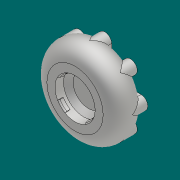
# Autodesk Inventor part: finger5
Saved by Autodesk Inventor 2018.2 (Build 222227000, 227)
## iProperties
Created: 2020-12-02
Part Number: finger5
Material: アルミニウム 6061
Document SubType Name: Modeling
Designer: gisen
Density: 2.7 g/cm^3
Appearance: アルミニウム - フラット
Author: gisen
Autodesk Inventor part; units mm, degrees
ref_plane "YZ Plane" through (0, 0, 0) normal (1, 0, 0) x (0, 1, 0)
ref_plane "XZ Plane" through (0, 0, 0) normal (0, 1, 0) x (-1, 0, 0)
ref_plane "XY Plane" through (0, 0, 0) normal (0, 0, 1) x (1, 0, 0)
sketch "スケッチ1" plane through (0, 0, 0) normal (0, 0, 1) x (1, 0, 0)
  line L0 (0, 0) -> (3.75, 0) construction
  line L1 (3.75, 0) -> (3.75, 1.7) construction
  line L2 (3.75, 1.7) -> (0, 1.7) construction
  line L3 (0, 1.7) -> (0, 0) construction
  line L4 (2.85, 1.7) -> (3.75, 0.8) construction
  line L5 (0, 4.7) -> (5.25, 4.7) construction
  arc A0 (5.25, -0.8) -> (5.25, 4.7) centre (5.25, 1.95) ccw
  line L6 (5.25, 4.7) -> (5.25, -0.8) construction
  arc A1 (3.75, 0) -> (3.75, -0.8) centre (4.05, -0.4) ccw construction
  line L7 (3.75, -0.8) -> (5.25, -0.8)
  line L8 (4.05, -0.4) -> (3.55, -0.4) construction
  line L9 (5.25, 1.95) -> (8, 1.95) construction
  line L10 (0, 4.7) -> (0, 1.7) construction
  line L11 (0, 1.7) -> (2.85, 1.7)
  line L12 (2.85, 1.7) -> (3.75, 0.8)
  line L13 (3.75, 0.8) -> (3.75, 0)
  line L14 (0, 1.7) -> (0, 2.7)
  line L15 (5.25, 4.7) -> (4.25, 4.7)
  arc A2 (0, 2.7) -> (4.25, 4.7) centre (0, 8.2156) ccw
  arc A3 (3.567, -0.5294) -> (3.75, -0.8) centre (4.05, -0.4) ccw
  line L16 (3.567, -0.5294) -> (3.4252, 0)
  line L17 (3.75, 0) -> (3.4252, 0)
  point P0 (3.8, -0.4)
  dimension "d0" = 1.7
  dimension "d1" = 3.75
  dimension "d2" = 45
  dimension "d3" = 0.8
  dimension "d4" = 3
  dimension "d5" = 5.5
  dimension "d6" = 0.8
  dimension "d7" = 0.4
  dimension "d8" = 0.2
  dimension "d9" = 8
  dimension "d25" = 1
  dimension "d26" = 2
  dimension "d27" = 75
  dimension "d30" = 90
  dimension "d33" = 0.3248
  constraints: 36 end point, 12 point on circle, 6 point on line, 4 centre point, 4 horizontal, 2 midpoint, 2 parallel, 2 tangent, 1 coincident, 1 concentric, 1 horizontal alignment, 1 perpendicular
  measures "d0" distance between parallel lines of L0 L2
  measures "d1" distance between parallel lines of L3 L1
  measures "d2" angle of L4 L2
  measures "d3" distance of L0.end L4.end
  measures "d4" distance between parallel lines of L2 L5
  measures "d5" distance of L5.end L6.end
  measures "d6" distance from line of L6.end L0
  measures "d7" distance from line of L7 L8.start
  measures "d8" distance from line of L8.end L1
  measures "d9" distance from line of L3 L9.end
  measures "d25" distance from line of L6 L15.end
  measures "d26" distance from line of L5 L14.end
  measures "d27" angle of L17 L16
  measures "d30" angle of L1 L17
  measures "d33" distance from line of L1 L16.end
revolve "回転1" add sketch "スケッチ1" angle 360 about axis through (0, 4.7, 0) along (0, -1, 0)
sketch "スケッチ2" plane through (0, -0.8, 0) normal (0, -1, 0) x (1, 0, 0)
  circle A0 centre (0, 0) radius 3.85 construction
  line L0 (0, 0) -> (1.925, -3.3342)
  line L1 (0, 0) -> (-1.925, -3.3342)
  arc A1 (-1.925, -3.3342) -> (1.925, -3.3342) centre (0, 0) ccw
  line L2 (0, 0) -> (0, -3.85) construction
  line L3 (0, 0) -> (3.3342, 1.925)
  line L4 (0, 0) -> (3.3342, -1.925)
  arc A2 (3.3342, -1.925) -> (3.3342, 1.925) centre (0, 0) ccw
  line L5 (0, 0) -> (3.85, 0) construction
  line L6 (0, 0) -> (-1.925, 3.3342)
  line L7 (0, 0) -> (1.925, 3.3342)
  arc A3 (1.925, 3.3342) -> (-1.925, 3.3342) centre (0, 0) ccw
  line L8 (0, 0) -> (0, 3.85) construction
  line L9 (0, 0) -> (-3.3342, -1.925)
  line L10 (0, 0) -> (-3.3342, 1.925)
  arc A4 (-3.3342, 1.925) -> (-3.3342, -1.925) centre (0, 0) ccw
  line L11 (0, 0) -> (-3.85, 0) construction
  point P0 (0, 0)
  point P1 (0, 0)
  point P2 (0, 0)
  dimension "d11" = 60
  dimension "d12" = 30
  dimension "d15" = 360
  constraints: 24 end point, 14 point on circle, 6 coincident, 4 centre point, 1 vertical, 39 other
  measures "d11" angle of L1 L0
  measures "d12" angle of L2 L0
extrude "押し出し1" cut sketch "スケッチ2" against normal blind 0.8
sketch "スケッチ3" plane through (0, 4.7, 0) normal (0, 1, 0) x (1, 0, 0)
  line L0 (-4.8163, 0) -> (-6.75, 0) construction
  line L1 (-4.8163, 1.25) -> (-6.75, 1.25)
  line L2 (-6.75, -1.25) -> (-4.8163, -1.25)
  arc A0 (-6.75, 1.25) -> (-6.75, -1.25) centre (-6.75, 0) ccw
  circle A1 centre (0, 0) radius 8 construction
  arc A2 (-4.8163, 1.25) -> (-4.8163, -1.25) centre (0, 0) ccw
  point P0 (-5.7831, 0)
  dimension "d19" = 1.25
  constraints: 8 end point, 4 point on circle, 3 tangent, 2 centre point, 1 coincident, 1 horizontal, 1 midpoint, 1 parallel, 1 point on line
  measures "d19" radius of A0
extrude "押し出し2" add sketch "スケッチ3" against normal blind 2.75
pattern_circular "円形状パターン1" count 8 over 360 about axis through (0, 0.4, 0) along (0, -1, 0) of "押し出し2"
sketch "スケッチ4" plane through (0, -0.8, 0) normal (0, -1, 0) x (1, 0, 0)
  arc A0 (1.875, 3.2476) -> (-1.875, 3.2476) centre (0, 0) ccw projected
  line L0 (1.925, 3.3342) -> (1.875, 3.2476) projected
  arc A1 (1.925, 3.3342) -> (-1.925, 3.3342) centre (0, 0) ccw projected
  line L1 (-1.875, 3.2476) -> (-1.925, 3.3342) projected
  arc A2 (3.2476, -1.875) -> (3.2476, 1.875) centre (0, 0) ccw projected
  line L2 (3.3342, -1.925) -> (3.2476, -1.875) projected
  arc A3 (3.3342, -1.925) -> (3.3342, 1.925) centre (0, 0) ccw projected
  line L3 (3.2476, 1.875) -> (3.3342, 1.925) projected
  arc A4 (-1.875, -3.2476) -> (1.875, -3.2476) centre (0, 0) ccw projected
  line L4 (-1.925, -3.3342) -> (-1.875, -3.2476) projected
  arc A5 (-1.925, -3.3342) -> (1.925, -3.3342) centre (0, 0) ccw projected
  line L5 (1.875, -3.2476) -> (1.925, -3.3342) projected
  arc A6 (-3.2476, 1.875) -> (-3.2476, -1.875) centre (0, 0) ccw projected
  line L6 (-3.3342, 1.925) -> (-3.2476, 1.875) projected
  arc A7 (-3.3342, 1.925) -> (-3.3342, -1.925) centre (0, 0) ccw projected
  line L7 (-3.2476, -1.875) -> (-3.3342, -1.925) projected
extrude "押し出し3" add sketch "スケッチ4" against normal up to surface (0.8 mm away)
sketch "スケッチ5" plane through (-6.75, 4.7, -1.25) normal (0, 1, 0) x (1, 0, 0)
  arc A0 (4.0283, -5.7394) -> (5.5, -6.349) centre (6.75, -1.25) ccw projected
  line L0 (5.5, -6.349) -> (5.5, -8) projected
  arc A1 (5.5, -8) -> (8, -8) centre (6.75, -8) ccw projected
  line L1 (8, -8) -> (8, -6.349) projected
  arc A2 (8, -6.349) -> (9.4717, -5.7394) centre (6.75, -1.25) ccw projected
  line L2 (9.4717, -5.7394) -> (10.6391, -6.9069) projected
  arc A3 (10.6391, -6.9069) -> (12.4069, -5.1391) centre (11.523, -6.023) ccw projected
  line L3 (12.4069, -5.1391) -> (11.2394, -3.9717) projected
  arc A4 (11.2394, -3.9717) -> (11.849, -2.5) centre (6.75, -1.25) ccw projected
  line L4 (11.849, -2.5) -> (13.5, -2.5) projected
  arc A5 (13.5, -2.5) -> (13.5, 0) centre (13.5, -1.25) ccw projected
  line L5 (13.5, 0) -> (11.849, 0) projected
  arc A6 (11.849, 0) -> (11.2394, 1.4717) centre (6.75, -1.25) ccw projected
  line L6 (11.2394, 1.4717) -> (12.4069, 2.6391) projected
  arc A7 (12.4069, 2.6391) -> (10.6391, 4.4069) centre (11.523, 3.523) ccw projected
  line L7 (10.6391, 4.4069) -> (9.4717, 3.2394) projected
  arc A8 (9.4717, 3.2394) -> (8, 3.849) centre (6.75, -1.25) ccw projected
  line L8 (8, 3.849) -> (8, 5.5) projected
  arc A9 (8, 5.5) -> (5.5, 5.5) centre (6.75, 5.5) ccw projected
  line L9 (5.5, 5.5) -> (5.5, 3.849) projected
  arc A10 (5.5, 3.849) -> (4.0283, 3.2394) centre (6.75, -1.25) ccw projected
  line L10 (4.0283, 3.2394) -> (2.8609, 4.4069) projected
  arc A11 (2.8609, 4.4069) -> (1.0931, 2.6391) centre (1.977, 3.523) ccw projected
  line L11 (1.0931, 2.6391) -> (2.2606, 1.4717) projected
  arc A12 (2.2606, 1.4717) -> (1.651, 0) centre (6.75, -1.25) ccw projected
  line L12 (1.651, 0) -> (0, 0) projected
  arc A13 (0, 0) -> (0, -2.5) centre (0, -1.25) ccw projected
  line L13 (0, -2.5) -> (1.651, -2.5) projected
  arc A14 (1.651, -2.5) -> (2.2606, -3.9717) centre (6.75, -1.25) ccw projected
  line L14 (2.2606, -3.9717) -> (1.0931, -5.1391) projected
  arc A15 (1.0931, -5.1391) -> (2.8609, -6.9069) centre (1.977, -6.023) ccw projected
  line L15 (2.8609, -6.9069) -> (4.0283, -5.7394) projected
  circle A16 centre (6.75, -1.25) radius 4.25 projected
extrude "押し出し4" add sketch "スケッチ5" along normal blind 0.1
fillet "フィレット1" radius 1 16 edges at (2.7217, 4.75, -4.4894) (1.25, 4.75, -5.099) (-1.25, 4.75, -5.099) (-2.7217, 4.75, -4.4894) (-4.4894, 4.75, -2.7217) (-5.099, 4.75, -1.25) (-5.099, 4.75, 1.25) (-4.4894, 4.75, 2.7217) (-2.7217, 4.75, 4.4894) (-1.25, 4.75, 5.099) (1.25, 4.75, 5.099) (2.7217, 4.75, 4.4894) (4.4894, 4.75, 2.7217) (5.099, 4.75, 1.25) (5.099, 4.75, -1.25) (4.4894, 4.75, -2.7217)
equation "\"d7\" = 0.5 * d6"
equation "\"d12\" = 0.5 * d11"
